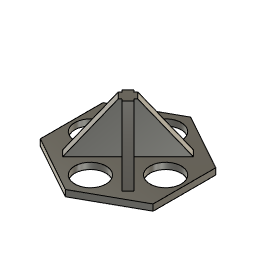
conductive_015mm_hexagon_loose (Autodesk Fusion 360 design; units mm, degrees)
Autodesk Fusion 360 part; units mm, degrees
other "Base Mesh Feature1"
sketch "Sketch1" plane through (0, 0, 0) normal (0, 0, 1) x (1, 0, 0)
  circle A0 centre (0, 0) radius 10
  dimension "d1" = 20
  constraint coincident A0.centre origin
  measures "d1" diameter of A0
other "Modify1"
sketch "Sketch2" plane through (0, 0, 0) normal (0, 0, 1) x (1, 0, 0)
  line L0 (18, 20) -> (20, 20)
  line L1 (18, -10) -> (18, 10)
  line L2 (-18, 10) -> (0, 20)
  line L3 (18, 10) -> (0, 20)
  line L4 (0, -20) -> (18, -10)
  line L5 (0, -20) -> (-18, -10)
  line L6 (-18, 10) -> (-18, -10)
  line L7 (0, 22) -> (0, -22) construction
  line L8 (-20, 0) -> (20, 0) construction
  line L9 (0, 12) -> (-19, 12) construction
  circle A0 centre (0, 12) radius 4.9927
  circle A1 centre (-12, 0) radius 4.9927
  circle A2 centre (0, -12) radius 4.9927
  circle A3 centre (12, 0) radius 4.9927
  line L10 (0, 0) -> (20, 20) construction
  dimension "d5" = 360
  constraint horizontal L0
  constraint perpendicular L0 L1
  constraint parallel L2 L4
  constraint parallel L3 L5
  constraint vertical L7
  constraint perpendicular L1 L8
  constraint coincident L7 L9.start
  constraint perpendicular L7 L9
  constraint coincident L9.start A0.centre
  constraint coincident L10.start origin
extrude "Extrude1" add sketch "Sketch2" along normal blind 2 contours L1 L2 L3 L4 L5 L6 | A0 | A1 | A2 | A3 makes body 1
extrude "Extrude2" cut sketch "Sketch2" along normal blind 7 contours A0 | A1 | A2 | A3 bodies 1
ref_plane "WorkPlane1" through (10, 10, 0) normal (0.707107, -0.707107, 0) x (0.707107, 0.707107, 0)
sketch "Sketch3" plane through (0, 0, 0) normal (0.707107, -0.707107, 0) x (0.707107, 0.707107, 0)
  line L0 (-15, 2) -> (0, 2)
  line L1 (0, 18) -> (-2.1955, 18)
  line L2 (-2.1955, 18) -> (-14.7632, 2)
  line L3 (0, 18) -> (2.1955, 18)
  line L4 (2.1955, 18) -> (14.7632, 2)
  line L5 (15, 2) -> (0, 2)
  constraint horizontal L0
  constraint horizontal L1
  constraint coincident L0 L2.end
extrude "Extrude3" add sketch "Sketch3" along normal mid plane 2.72 separate body makes body 2
copy_body "CopyPasteBodies1" bodies 2 makes body 3
move_body "Move1" bodies 3 to x (0, -1, 0) y (1, 0, 0) z (0, 0, 1) at (0, 0, 0)
combine "Combine1" operation add target body 2 tool bodies 3 1
